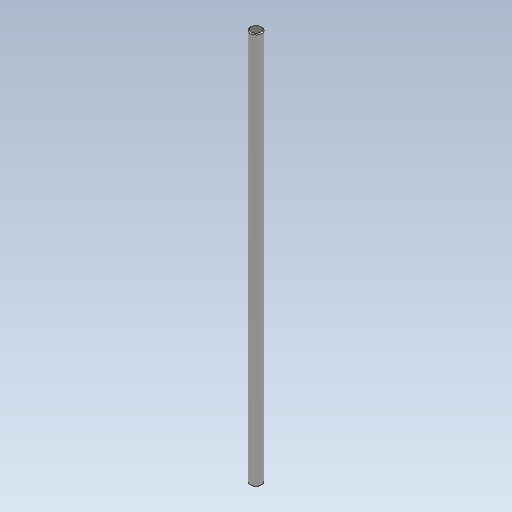
# Autodesk Inventor part: shaft
Saved by Autodesk Inventor 2020.2 (Build 242310000, 310)
## iProperties
Created: 2020-03-23
Part Number: shaft
Material: Stainless Steel
Document SubType Name: Modeling
Designer: agmle
Density: 8 g/cm^3
Appearance: Semi-Polished
Mass: 6.87112 g
Surface Area: 10.9553 cm^2
Volume: 0.85889 cm^3
Author: agmle
Autodesk Inventor part; units mm, degrees
ref_plane "YZ Plane" through (0, 0, 0) normal (1, 0, 0) x (0, 1, 0)
ref_plane "XZ Plane" through (0, 0, 0) normal (0, 1, 0) x (-1, 0, 0)
ref_plane "XY Plane" through (0, 0, 0) normal (0, 0, 1) x (1, 0, 0)
sketch "Sketch1" plane through (0, 0, 0) normal (0, 1, 0) x (-1, 0, 0)
  circle A0 centre (0, 0) radius 1.5875
  dimension "d0" = 3.175
  constraints: 1 centre point, 1 coincident
  measures "d0" diameter of A0
extrude "Extrusion1" add sketch "Sketch1" along normal blind 108.5596
chamfer "Chamfer1" distance 0.254 angle 45 2 edges at (1.5875, 0, 0) (1.5875, 108.5596, 0)
body "Solid1"
